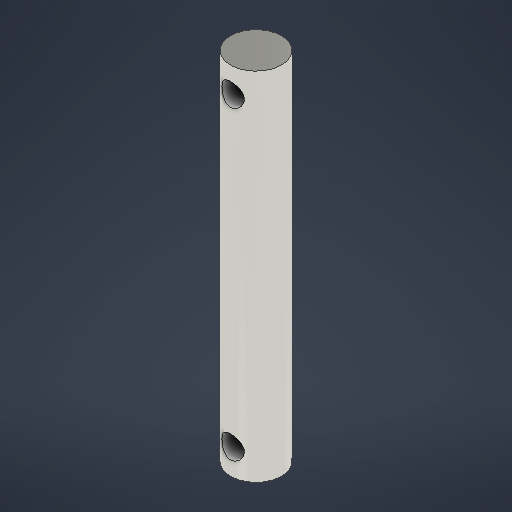
# Autodesk Inventor part: short_tibia
Saved by Autodesk Inventor 2027.1 (Build 311270010, 270A)
## iProperties
Created: 2026-08-17
Part Number: short_tibia
Material: Ogólny
Document SubType Name: Modeling
Designer: User
Density: 1 g/cm^3
Appearance: Domyślna
Author: User
Autodesk Inventor part; units mm, degrees
ref_plane "YZ Plane" through (0, 0, 0) normal (1, 0, 0) x (0, 1, 0)
ref_plane "XZ Plane" through (0, 0, 0) normal (0, 1, 0) x (-1, 0, 0)
ref_plane "XY Plane" through (0, 0, 0) normal (0, 0, 1) x (1, 0, 0)
sketch "Szkic1" plane through (0, 0, 0) normal (0, 1, 0) x (-1, 0, 0)
  circle A0 centre (0, 0) radius 5
  dimension "d0" = 10
  constraints: 1 centre point, 1 coincident
  measures "d0" diameter of A0
extrude "Wyciągnięcie proste1" add sketch "Szkic1" along normal blind 70
sketch "Szkic2" plane through (0, 0, 0) normal (0, 0, 1) x (1, 0, 0)
  line L0 (0, 0) -> (0, 5)
  circle A0 centre (0, 5) radius 2.2
  line L1 (5, 70) -> (-5, 70) projected
  line L2 (0, 70) -> (0, 65)
  circle A1 centre (0, 65) radius 2.2
  dimension "d3" = 5
  dimension "d4" = 4.4
  dimension "d7" = 5
  dimension "d8" = 4.4
  constraints: 4 end point, 2 centre point, 2 coincident, 2 vertical, 1 midpoint
  measures "d3" distance of L0.start L0.end
  measures "d4" diameter of A0
  measures "d7" distance of L2.start L2.end
  measures "d8" diameter of A1
extrude "Wyciągnięcie proste2" cut sketch "Szkic2" along normal mid plane 22.5
